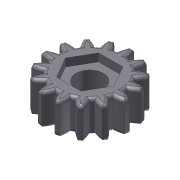
# Autodesk Inventor part: Engranaje_varilla_Z
Saved by Autodesk Inventor 2015 SP2 (Build 190223200, 223)
## iProperties
Created: 2015-05-13
Material: Steel
Document SubType Name: Modeling
Designer: E.Beroiz
Categories: <?xml version="1.0" encoding="UTF-16"?> <MemberInstance><Categories><FamilyTemplate><FamilyTemplateParameter ValueType="xs:double" Id="1" ObjectReferenceKey="da_z" ObjectType="kUserParameterObject"/><FamilyTemplateParameter ValueType="xs:double" Id="2" ObjectReferenceKey="da_b" ObjectType="kUserParameterObject"/><FamilyTemplateParameter ValueType="xs:double" Id="3" ObjectReferenceKey="da_beta" ObjectType="kUserParameterObject"/><FamilyTemplateParameter ValueType="xs:double" Id="4" ObjectReferenceKey="da_da" ObjectType="kUserParameterObject"/><FamilyTemplateParameter ValueType="xs:double" Id="5" ObjectReferenceKey="da_aw" ObjectType="kUserParameterObject"/><FamilyTemplateParameter ValueType="xs:string" Id="6" ObjectReferenceKey="EAIAABAAAACIAQAAAAAAAIAAAAAAAAAA" ObjectType="83910656" SubObjectId="SurfaceGeometry"/></FamilyTemplate><ParamToTemplateMap><ParamToTemplate CategoryParameter="//CategoryParameter[@InternalName='046C89C9-8512-4d59-83FE-43B91F4F132A']" TemplateParameter="1"/><ParamToTemplate CategoryParameter="//CategoryParameter[@InternalName='2552DF32-E462-4b46-AEBF-C6C7768E72AC']" TemplateParameter="2"/><ParamToTemplate CategoryParameter="//CategoryParameter[@InternalName='C9EE641D-15FC-4fae-A226-E94C4372FDD7']" TemplateParameter="3"/><ParamToTemplate><ParamToTemplate CategoryParameter="//CategoryParameter[@InternalName='00B6519A-459B-49c7-AD84-2E56D39A5744']" ConstantValue="-0.439000"/></ParamToTemplate><ParamToTemplate><ParamToTemplate CategoryParameter="//CategoryParameter[@InternalName='04B31F0E-C7A6-4894-AA32-9629BEFACF47']" ConstantValue="0.800000"/></ParamToTemplate><ParamToTemplate><ParamToTemplate CategoryParameter="//CategoryParameter[@InternalName='43CBEC2E-7847-49e7-A936-2F7889FCB2D9']" ConstantValue="0.300000"/></ParamToTemplate><ParamToTemplate><ParamToTemplate CategoryParameter="//CategoryParameter[@InternalName='B1EFC894-105D-4ebd-86BF-FA20ED196853']" ConstantValue="0.151900"/></ParamToTemplate><ParamToTemplate><ParamToTemplate CategoryParameter="//CategoryParameter[@InternalName='51175063-3D10-4879-93E8-6246FE8B403D']" ConstantValue="2060000000.000000"/></ParamToTemplate><ParamToTemplate><ParamToTemplate CategoryParameter="//CategoryParameter[@InternalName='A3A52E27-4454-46a9-B0BD-C932399B70AF']" ConstantValue="0.300000"/></ParamToTemplate><ParamToTemplate><ParamToTemplate CategoryParameter="//CategoryParameter[@InternalName='91B76062-C214-41d9-B1B9-14D2AB99603D']" ConstantValue="0.175000"/></ParamToTemplate><ParamToTemplate><ParamToTemplate CategoryParameter="//CategoryParameter[@InternalName='374E806E-8B8A-4dda-A9AA-1039D6500AD2']" ConstantValue="5.714286"/></ParamToTemplate><ParamToTemplate><ParamToTemplate CategoryParameter="//CategoryParameter[@InternalName='2D373A89-B862-43d6-8D0B-0CBF12AB9F6C']" ConstantValue="0.349066"/></ParamToTemplate><ParamToTemplate CategoryParameter="//CategoryParameter[@InternalName='37777632-D6A2-4fac-9D53-DB8ACD95C989']" TemplateParameter="4"/><ParamToTemplate CategoryParameter="//CategoryParameter[@InternalName='FD1017F1-B727-4f7e-9707-0F86F1FF9423']" TemplateParameter="5"/><ParamToTemplate><ParamToTemplate CategoryParameter="//CategoryParameter[@InternalName='9E1B4470-B2D3-4ff1-B813-535BB4CDF51A']" ConstantValue="3520000.000000"/></ParamToTemplate><ParamToTemplate><ParamToTemplate CategoryParameter="//CategoryParameter[@InternalName='F8452263-BFF6-458c-9FB1-07C4B99E95CD']" ConstantValue="11400000.000000"/></ParamToTemplate><ParamToTemplate><ParamToTemplate CategoryParameter="//CategoryParameter[@InternalName='3E3BB259-FD49-497f-8171-6EBC954A3479']" ConstantValue="2.000000"/></ParamToTemplate><ParamToTemplate CategoryParameter="//CategoryParameter[@InternalName='27C3BAF2-7550-4e4b-AE2C-0DB134B7D9B7']" TemplateParameter="6"/></ParamToTemplateMap><Category DisplayName="Gear" InternalName="DC85795E-93AB-48d5-8EEE-5A27447B64BD" Mnemonic="Gear"><CategoryParameter DisplayName="z" InternalName="046C89C9-8512-4d59-83FE-43B91F4F132A" Mnemonic="z"/><CategoryParameter DisplayName="b" InternalName="2552DF32-E462-4b46-AEBF-C6C7768E72AC" Mnemonic="b"/><CategoryParameter DisplayName="||b|" InternalName="C9EE641D-15FC-4fae-A226-E94C4372FDD7" Mnemonic="beta"/><CategoryParameter DisplayName="x" InternalName="00B6519A-459B-49c7-AD84-2E56D39A5744" Mnemonic="x"/><CategoryParameter DisplayName="a*" InternalName="04B31F0E-C7A6-4894-AA32-9629BEFACF47" Mnemonic="a"/><CategoryParameter DisplayName="c*" InternalName="43CBEC2E-7847-49e7-A936-2F7889FCB2D9" Mnemonic="c"/><CategoryParameter DisplayName="r|.f|*" InternalName="B1EFC894-105D-4ebd-86BF-FA20ED196853" Mnemonic="rf"/><CategoryParameter DisplayName="E" InternalName="51175063-3D10-4879-93E8-6246FE8B403D" Mnemonic="E"/><CategoryParameter DisplayName="||m|" InternalName="A3A52E27-4454-46a9-B0BD-C932399B70AF" Mnemonic="mi"/><Category DisplayName="SpurGear" InternalName="26C5A22E-A91E-4dfd-A3B3-23CCAFAE1764" Mnemonic="SpurGear"><CategoryParameter DisplayName="m" InternalName="91B76062-C214-41d9-B1B9-14D2AB99603D" Mnemonic="m"/><CategoryParameter DisplayName="P" InternalName="374E806E-8B8A-4dda-A9AA-1039D6500AD2" Mnemonic="PP"/><CategoryParameter DisplayName="||a|" InternalName="2D373A89-B862-43d6-8D0B-0CBF12AB9F6C" Mnemonic="alpha"/><CategoryParameter DisplayName="d|.a|" InternalName="37777632-D6A2-4fac-9D53-DB8ACD95C989" Mnemonic="da"/><CategoryParameter DisplayName="a|.w|" InternalName="FD1017F1-B727-4f7e-9707-0F86F1FF9423" Mnemonic="aw"/><CategoryParameter DisplayName="||s||.Flim|" InternalName="9E1B4470-B2D3-4ff1-B813-535BB4CDF51A" Mnemonic="sFlim"/><CategoryParameter DisplayName="||s||.Hlim|" InternalName="F8452263-BFF6-458c-9FB1-07C4B99E95CD" Mnemonic="sHlim"/><CategoryParameter DisplayName="tipo" InternalName="3E3BB259-FD49-497f-8171-6EBC954A3479" Mnemonic="type"/><CategoryParameter DisplayName="PitchDiameter" InternalName="27C3BAF2-7550-4e4b-AE2C-0DB134B7D9B7" Mnemonic="IDS_PITCHDIAM"/></Category></Category></Categories></MemberInstance>
Density: 1 g/cm^3
Appearance: Steel
Description: Cycl_engranajeVarillaZ
CustomPartVersion: 1
Author: E.Beroiz
Autodesk Inventor part; units mm, degrees
sketch "Sketch1" plane through (0, 0, 0) normal (0, 0, 1) x (1, 0, 0)
  circle A0 centre (0, 0) radius 13.4
  dimension "d0" = 26.8
  constraints: 1 centre point
  measures "d0" diameter of A0
extrude "Extrusion1" add sketch "Sketch1" along normal blind 10
ref_plane "Work Plane2" through (0, 0, 5) normal (0, 0, 1) x (1, 0, 0)
sketch "Sketch2" plane through (0, 0, 0) normal (0, 0, -1) x (-1, 0, 0)
  circle A0 centre (0, 0) radius 13.4 projected
  circle A1 centre (0, 0) radius 12.3913
  dimension "d3" = 24.7826
  constraints: 1 centre point, 1 coincident
  measures "d3" diameter of A1
surface extrude "Diámetro de separación" sketch "Sketch2" against normal through all shown no curves A1
ref_plane "Work Plane8" through (0, 0, 0) normal (0.9781476, 0.2079117, 0) x (0, 0, 1)
ref_plane "Work Plane9" through (0, 0, 0) normal (1, 0, 0) x (0, 1, 0)
spur gear teeth "Engranaje recto" teeth 15 pitch diameter 26.25 tip diameter 26.8 root diameter 20.8635 face width 10 start plane through (0, 0, 0) normal (0, 0, -1) x (-1, 0, 0)
sketch "Boceto4" plane through (0, 0, 10) normal (0, 0, 1) x (1, 0, 0)
  line L0 (7.7365, 0) -> (3.8682, -6.7)
  line L1 (3.8682, -6.7) -> (-3.8682, -6.7)
  line L2 (-3.8682, -6.7) -> (-7.7365, 0)
  line L3 (-7.7365, 0) -> (-3.8682, 6.7)
  line L4 (-3.8682, 6.7) -> (3.8682, 6.7)
  line L5 (3.8682, 6.7) -> (7.7365, 0)
  point P0 (0, 0)
  point P1 (0, 0)
  dimension "d52" = 13.4
  constraints: 12 end point, 1 coincident, 1 horizontal, 13 other
  measures "d52" distance between parallel lines of L4 L1
extrude "Extrusión3" cut sketch "Boceto4" against normal blind 2.5
sketch "Boceto5" plane through (0, 0, 7.5) normal (0, 0, 1) x (1, 0, 0)
  circle A0 centre (0, 0) radius 4.35
  dimension "d55" = 8.7
  constraints: 1 centre point, 1 coincident
  measures "d55" diameter of A0
extrude "Extrusión4" cut sketch "Boceto5" against normal through all
fillet "Empalme1" radius 1 60 edges at (-6.0243, 10.3263, 10) (-6.1316, 8.4395, 10) (-7.9593, 8.9204, 10) (-9.9581, 8.9664, 10) (-9.7035, 6.9832, 10) (-9.0342, 5.2159, 10) (-10.8994, 4.9119, 10) (-12.7442, 4.1408, 10) (-11.705, 2.4327, 10) (-10.3746, 1.0904, 10) (-11.955, 0.0541, 10) (-13.3266, -1.4007, 10) (-11.6825, -2.5384, 10) (-9.9212, -3.2236, 10) (-10.9434, -4.8131, 10) (-11.6047, -6.7, 10) (-9.64, -7.0707, 10) (-7.7523, -6.9802, 10) (-8.0396, -8.8481, 10) (-7.8763, -10.8408, 10) (-5.9307, -10.3803, 10) (-4.243, -9.5299, 10) (-3.7457, -11.3532, 10) (-2.786, -13.1072, 10) (-1.1959, -11.8951, 10) (0, -10.4317, 10) (1.1959, -11.8951, 10) (2.786, -13.1072, 10) (3.7457, -11.3532, 10) (4.243, -9.5299, 10) (5.9307, -10.3803, 10) (7.8763, -10.8408, 10) (8.0396, -8.8481, 10) (7.7523, -6.9802, 10) (9.64, -7.0707, 10) (11.6047, -6.7, 10) (10.9434, -4.8131, 10) (9.9212, -3.2236, 10) (11.6825, -2.5384, 10) (13.3266, -1.4007, 10) (11.955, 0.0541, 10) (10.3746, 1.0904, 10) (11.705, 2.4327, 10) (12.7442, 4.1408, 10) (10.8994, 4.9119, 10) (9.0342, 5.2159, 10) (9.7035, 6.9832, 10) (9.9581, 8.9664, 10) (7.9593, 8.9204, 10) (6.1316, 8.4395, 10) (6.0243, 10.3263, 10) (5.4503, 12.2415, 10) (3.6429, 11.3866, 10) (2.1689, 10.2038, 10) (1.3034, 11.8838, 10) (0, 13.4, 10) (-1.3034, 11.8838, 10) (-2.1689, 10.2038, 10) (-3.6429, 11.3866, 10) (-5.4503, 12.2415, 10)
fillet "Empalme2" radius 1 60 edges at (-6.0243, 10.3263, 0) (-5.4503, 12.2415, 0) (-3.6429, 11.3866, 0) (-2.1689, 10.2038, 0) (-1.3034, 11.8838, 0) (0, 13.4, 0) (1.3034, 11.8838, 0) (2.1689, 10.2038, 0) (3.6429, 11.3866, 0) (5.4503, 12.2415, 0) (6.0243, 10.3263, 0) (6.1316, 8.4395, 0) (7.9593, 8.9204, 0) (9.9581, 8.9664, 0) (9.7035, 6.9832, 0) (9.0342, 5.2159, 0) (10.8994, 4.9119, 0) (12.7442, 4.1408, 0) (11.705, 2.4327, 0) (10.3746, 1.0904, 0) (11.955, 0.0541, 0) (13.3266, -1.4007, 0) (11.6825, -2.5384, 0) (9.9212, -3.2236, 0) (10.9434, -4.8131, 0) (11.6047, -6.7, 0) (9.64, -7.0707, 0) (7.7523, -6.9802, 0) (8.0396, -8.8481, 0) (7.8763, -10.8408, 0) (5.9307, -10.3803, 0) (4.243, -9.5299, 0) (3.7457, -11.3532, 0) (2.786, -13.1072, 0) (1.1959, -11.8951, 0) (0, -10.4317, 0) (-1.1959, -11.8951, 0) (-2.786, -13.1072, 0) (-3.7457, -11.3532, 0) (-4.243, -9.5299, 0) (-5.9307, -10.3803, 0) (-7.8763, -10.8408, 0) (-8.0396, -8.8481, 0) (-7.7523, -6.9802, 0) (-9.64, -7.0707, 0) (-11.6047, -6.7, 0) (-10.9434, -4.8131, 0) (-9.9212, -3.2236, 0) (-11.6825, -2.5384, 0) (-13.3266, -1.4007, 0) (-11.955, 0.0541, 0) (-10.3746, 1.0904, 0) (-11.705, 2.4327, 0) (-12.7442, 4.1408, 0) (-10.8994, 4.9119, 0) (-9.0342, 5.2159, 0) (-9.7035, 6.9832, 0) (-9.9581, 8.9664, 0) (-7.9593, 8.9204, 0) (-6.1316, 8.4395, 0)
fillet "Empalme3" radius 1 1 edges at (-4.35, 0, 0)
equation "\"d0\" = da_da"
equation "\"d1\" = da_b"
equation "\"d3\" = da_dw"
equation "\"d16\" = da_aw"
equation "\"d43\" = da_aw"
equation "\"d46\" = da_aw"
equation "\"da_da\" = 26.8"
equation "\"da_b\" = 10"
equation "\"da_dw\" = 24.782609"
equation "\"da_aw\" = 19"
body "Solid1"
body "Srf1"
